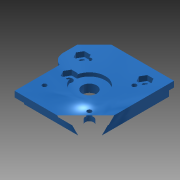
# Autodesk Inventor part: ExtruderSatoerMotorMount
Saved by Autodesk Inventor 2015 SP1 (Build 190203100, 203)
## iProperties
Created: 2015-05-03
Part Number: ExtruderSatoerMotorMount
Material: Generic
Document SubType Name: Modeling
Designer: Jack
Density: 1 g/cm^3
Appearance: Cyan
Author: Jack
Autodesk Inventor part; units mm, degrees
ref_plane "YZ Plane" through (0, 0, 0) normal (1, 0, 0) x (0, 1, 0)
ref_plane "XZ Plane" through (0, 0, 0) normal (0, 1, 0) x (-1, 0, 0)
ref_plane "XY Plane" through (0, 0, 0) normal (0, 0, 1) x (1, 0, 0)
sketch "Sketch1" plane through (0, 0, 0) normal (0, 0, 1) x (1, 0, 0)
  line L0 (0, 0) -> (45.5, 0)
  line L1 (45.5, 0) -> (45.5, 54.5)
  line L2 (0, 30.5) -> (-0.25, 30.5)
  line L3 (45.5, 54.5) -> (0, 54.5)
  line L4 (-5.4281, 33.75) -> (-8.7859, 33.3971)
  arc A0 (-9.25, 36.25) -> (-8.7859, 33.3971) centre (-0.25, 36.25) ccw
  arc A1 (-0.25, 57.75) -> (-9.25, 48.75) centre (-0.25, 48.75) ccw
  line L5 (-9.25, 48.75) -> (-9.25, 36.25)
  line L6 (0, 0) -> (0, 3)
  line L7 (0, 3) -> (-3.25, 3)
  line L8 (-3.25, 3) -> (-3.25, 16)
  line L9 (-3.25, 16) -> (0, 16)
  line L10 (0, 16) -> (0, 30.5)
  arc A2 (-5.4281, 33.75) -> (-0.25, 30.5) centre (-0.25, 36.25) ccw
  line L11 (0, 54.5) -> (0, 57.75)
  line L12 (0, 57.75) -> (-0.25, 57.75)
  dimension "d0" = 45.5
  dimension "d1" = 54.5
  dimension "d9" = 84
  dimension "d10" = 13
  dimension "d11" = 3
  dimension "d12" = 3.25
  dimension "d13" = 14.5
  dimension "d18" = 9
  dimension "d19" = 54.75
  dimension "d24" = 12.5
  dimension "d27" = 5.75
  dimension "d30" = 3.25
  dimension "d31" = 45.5
  dimension "d68" = 0.25
  dimension "d69" = 3.25
  constraints: 26 end point, 6 perpendicular, 6 point on circle, 4 tangent, 3 centre point, 3 vertical, 2 horizontal, 1 equal radius, 1 point on line, 1 vertical alignment
  measures "d0" distance of L0.start L0.end
  measures "d1" distance of L0.end L1.end
  measures "d9" angle of L5 L4
  measures "d10" distance of L7.end L8.end
  measures "d11" distance between parallel lines of L0 L7
  measures "d12" distance of L8.end L9.end
  measures "d13" distance of L9.end L2.start
  measures "d18" radius of A0
  measures "d19" distance between parallel lines of L1 L5
  measures "d24" distance of A1.centre A0.centre
  measures "d27" radius of A2
  measures "d30" distance of L3.end L11.end
  measures "d31" distance between parallel lines of L11 L1
  measures "d68" distance of L2.start L2.end
  measures "d69" vertical distance of L2.start L4.start
extrude "Extrusion1" add sketch "Sketch1" along normal blind 4
sketch "Sketch2" plane through (0, 0, 4) normal (0, 0, 1) x (1, 0, 0)
  line L0 (0, 0) -> (45.5, 0) projected
  line L1 (0, 57.75) -> (-0.25, 57.75) projected
  arc A0 (-0.25, 57.75) -> (-9.25, 48.75) centre (-0.25, 48.75) ccw projected
  line L2 (-9.25, 48.75) -> (-9.25, 36.25) projected
  arc A1 (-9.25, 36.25) -> (-8.7859, 33.3971) centre (-0.25, 36.25) ccw projected
  arc A2 (-5.4281, 33.75) -> (-0.25, 30.5) centre (-0.25, 36.25) ccw projected
  line L3 (-3.25, 16) -> (-3.25, 3) projected
  arc A3 (-9.25, 36.25) -> (-3.25, 27.7647) centre (-0.25, 36.25) ccw
  line L4 (0, 57.75) -> (48.75, 57.75)
  line L5 (48.75, 57.75) -> (48.75, -3.25)
  line L6 (48.75, -3.25) -> (-3.25, -3.25)
  line L7 (-3.25, 27.7647) -> (-3.25, -3.25)
  dimension "d32" = 48.75
  dimension "d33" = 61
  constraints: 9 end point, 3 point on circle, 2 horizontal, 2 point on line, 1 centre point, 1 coincident, 1 perpendicular
  measures "d32" distance of L1.start L4.end
  measures "d33" distance of L4.end L5.end
extrude "Extrusion2" add sketch "Sketch2" along normal blind 4
sketch "Sketch4" plane through (0, 0, 0) normal (0, 0, -1) x (-1, 0, 0)
  line L0 (-48.75, 57.75) -> (0, 57.75) projected
  line L1 (-48.75, -3.25) -> (-48.75, 57.75) projected
  point P0 (-37.75, 41.35)
  point P1 (-6.75, 41.35)
  point P2 (-37.75, 10.35)
  point P3 (-6.75, 10.35)
  dimension "d39" = 31
  dimension "d40" = 31
  dimension "d41" = 16.4
  dimension "d42" = 11
  constraints: 2 horizontal alignment, 2 vertical alignment
  measures "d39" distance of point (-6.75, 41.35) point (-37.75, 41.35)
  measures "d40" distance of point (-6.75, 10.35) point (-6.75, 41.35)
  measures "d41" distance from line of L0 point (-37.75, 41.35)
  measures "d42" distance from line of L1 point (-37.75, 41.35)
hole "Hole1" at (37.75, 41.35, 0) at (6.75, 41.35, 0) at (37.75, 10.35, 0) at (6.75, 10.35, 0) direction (0, 0, 1) diameter 3 end through all counterbore diameter 5.8 counterbore depth 3.2
sketch "Sketch5" plane through (0, 0, 8) normal (0, 0, 1) x (1, 0, 0)
  circle A0 centre (37.75, 10.35) radius 1.5 projected
  circle A1 centre (37.75, 41.35) radius 1.5 projected
  circle A2 centre (6.75, 41.35) radius 1.5 projected
  circle A3 centre (6.75, 10.35) radius 1.5 projected
  line L0 (6.75, 41.35) -> (37.75, 10.35) construction
  line L1 (37.75, 41.35) -> (6.75, 10.35) construction
  point P0 (0, 0)
  point P1 (22.25, 25.85)
  constraints: 4 end point, 1 midpoint
hole "Hole2" at (22.25, 25.85, 8) direction (0, 0, -1) diameter 10 end through all counterbore diameter 22 counterbore depth 2.5
sketch "Sketch6" plane through (0, 0, 0) normal (0, 0, -1) x (-1, 0, 0)
  circle A0 centre (-6.75, 41.35) radius 2.9 projected
  circle A1 centre (-6.75, 10.35) radius 2.9 projected
  circle A2 centre (-35.25, 48.25) radius 2.25 projected
  circle A3 centre (0.75, 40.85) radius 2.25 projected
  circle A4 centre (-5.85, 25.35) radius 2.25 projected
hole "Hole3" at (35.25, 48.25, 0) at (-0.75, 40.85, 0) at (5.85, 25.35, 0) direction (0, 0, 1) diameter 4.5 end through all
sketch "Sketch7" plane through (0, 0, 8) normal (0, 0, 1) x (1, 0, 0)
  circle A0 centre (-0.75, 40.85) radius 2.25 projected
  circle A1 centre (35.25, 48.25) radius 2.25 projected
  circle A2 centre (5.85, 25.35) radius 2.25 projected
  line L0 (3.5224, 40.85) -> (1.3862, 37.15)
  line L1 (1.3862, 37.15) -> (-2.8862, 37.15)
  line L2 (-2.8862, 37.15) -> (-5.0224, 40.85)
  line L3 (-5.0224, 40.85) -> (-2.8862, 44.55)
  line L4 (-2.8862, 44.55) -> (1.3862, 44.55)
  line L5 (1.3862, 44.55) -> (3.5224, 40.85)
  line L6 (39.5224, 48.25) -> (37.3862, 44.55)
  line L7 (37.3862, 44.55) -> (33.1138, 44.55)
  line L8 (33.1138, 44.55) -> (30.9776, 48.25)
  line L9 (30.9776, 48.25) -> (33.1138, 51.95)
  line L10 (33.1138, 51.95) -> (37.3862, 51.95)
  line L11 (37.3862, 51.95) -> (39.5224, 48.25)
  line L12 (10.1224, 25.35) -> (7.9862, 21.65)
  line L13 (7.9862, 21.65) -> (3.7138, 21.65)
  line L14 (3.7138, 21.65) -> (1.5776, 25.35)
  line L15 (1.5776, 25.35) -> (3.7138, 29.05)
  line L16 (3.7138, 29.05) -> (7.9862, 29.05)
  line L17 (7.9862, 29.05) -> (10.1224, 25.35)
  point P0 (0, 0)
  dimension "d64" = 7.4
  constraints: 36 end point, 3 coincident, 3 horizontal, 2 parallel, 39 other
  measures "d64" distance between parallel lines of L1 L4
extrude "Extrusion3" cut sketch "Sketch7" against normal blind 3.5
body "Solid1"
